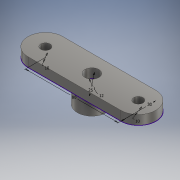
# Autodesk Inventor part: pr3defauldetail
Saved by Autodesk Inventor 2018 (Build 220112000, 112)
## iProperties
Created: 2020-04-08
Part Number: pr3defauldetail
Material: Нержавеющая сталь
Document SubType Name: Обычные детали
Designer: asus
Density: 8 g/cm^3
Appearance: С умеренной полировкой
Author: asus
Autodesk Inventor part; units mm, degrees
ref_plane "YZ Plane" through (0, 0, 0) normal (1, 0, 0) x (0, 1, 0)
ref_plane "XZ Plane" through (0, 0, 0) normal (0, 1, 0) x (-1, 0, 0)
ref_plane "XY Plane" through (0, 0, 0) normal (0, 0, 1) x (1, 0, 0)
sketch "Эскиз1" plane through (0, 0, 0) normal (0, 0, 1) x (1, 0, 0)
  line L0 (-40, 0) -> (40, 0) construction
  line L1 (-40, -15) -> (40, -15)
  line L2 (40, 15) -> (-40, 15)
  arc A0 (-40, 15) -> (-40, -15) centre (-40, 0) ccw
  arc A1 (40, -15) -> (40, 15) centre (40, 0) ccw
  circle A2 centre (0, 0) radius 12.5
  circle A3 centre (-40, 0) radius 5
  circle A4 centre (40, 0) radius 5
  circle A5 centre (0, 0) radius 6
  dimension "d1" = 30
  dimension "d2" = 80
  dimension "d5" = 25
  dimension "d6" = 10
  dimension "d7" = 10
  dimension "d8" = 12
  constraints: 8 end point, 6 centre point, 4 coincident, 4 point on circle, 4 tangent, 1 horizontal, 1 midpoint, 1 parallel
  measures "d1" diameter of A1
  measures "d2" distance of L0.start L0.end
  measures "d5" diameter of A2
  measures "d6" diameter of A3
  measures "d7" diameter of A4
  measures "d8" diameter of A5
extrude "Выдавливание1" add sketch "Эскиз1" along normal blind 8 contours A0 L2 A1 L1 | A2 | A3 | A4 | A5
hole "Отверстие1" at (40, 0, 0) direction (0, 0, 1) diameter 8 end through all
hole "Отверстие2" at (-40, 0, 0) direction (0, 0, 1) diameter 8 end through all
extrude "Выдавливание2" add sketch "Эскиз1" against normal blind 15 contours A2
extrude "Выдавливание3" cut sketch "Эскиз1" along normal blind 15 contours A5
equation "\"Радиус_гибки\" = Толщина"
equation "\"Ширина_просечки\" = Толщина"
equation "\"Глубина_просечки\" = 0.5 * Толщина"
equation "\"Размер_просечки\" = 4 * Толщина"
equation "\"Мин_остаток\" = 2 * Толщина"
equation "\"Радиус_перехода\" = Радиус_гибки"
equation "\"Радиус_Якоби\" = Толщина"
equation "\"Размер_зазора\" = Толщина"
equation "\"Толщина\" = 0.5"
